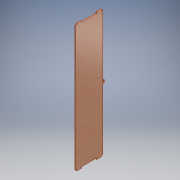
# Autodesk Inventor part: Frente_Controle
Saved by Autodesk Inventor 2017 (Build 210142000, 142)
## iProperties
Created: 2017-10-03
Part Number: Frente_Controle
Material: Wood (Oak)
Document SubType Name: Modeling
Designer: Felipe
Density: 0.76 g/cm^3
Appearance: White Oak - Natural Medium Gloss
Author: Felipe
Autodesk Inventor part; units mm, degrees
ref_plane "YZ Plane" through (0, 0, 0) normal (1, 0, 0) x (0, 1, 0)
ref_plane "XZ Plane" through (0, 0, 0) normal (0, 1, 0) x (-1, 0, 0)
sketch "Sketch1" plane through (0, 0, 0) normal (1, 0, 0) x (0, 1, 0)
  line L0 (0, 0) -> (195, 0) construction
  line L1 (195, 0) -> (195, -900)
  line L2 (195, -900) -> (0, -900) construction
  line L3 (0, -900) -> (0, 0)
  line L4 (195, -450) -> (0, -450) construction
  line L5 (186.046, 0) -> (151.046, 0) construction
  line L6 (151.046, 0) -> (151.046, 8.8542)
  line L7 (151.046, 8.8542) -> (186.046, 8.8542)
  line L8 (186.046, 8.8542) -> (186.046, 0)
  line L9 (43.046, 0) -> (8.046, 0) construction
  line L10 (8.046, 0) -> (8.046, 8.8542)
  line L11 (8.046, 8.8542) -> (43.046, 8.8542)
  line L12 (43.046, 8.8542) -> (43.046, 0)
  line L13 (151.046, 0) -> (43.046, 0)
  line L14 (8.046, 0) -> (0, 0)
  line L15 (186.046, 0) -> (195, 0)
  line L16 (0, -900) -> (195, -900) construction
  line L17 (186.046, -900) -> (151.046, -900) construction
  line L18 (151.046, -900) -> (151.046, -908.8542)
  line L19 (151.046, -908.8542) -> (186.046, -908.8542)
  line L20 (186.046, -908.8542) -> (186.046, -900)
  line L21 (43.046, -900) -> (8.046, -900) construction
  line L22 (8.046, -900) -> (8.046, -908.8542)
  line L23 (8.046, -908.8542) -> (43.046, -908.8542)
  line L24 (43.046, -908.8542) -> (43.046, -900)
  line L25 (151.046, -900) -> (43.046, -900)
  line L26 (8.046, -900) -> (0, -900)
  line L27 (186.046, -900) -> (195, -900)
  dimension "d0" = 900
  dimension "d1" = 195
  dimension "d2" = 35
  dimension "d3" = 108
  dimension "d4" = 8.046
  dimension "d5" = 8.954
  constraints: 56 end point, 8 symmetric about line, 6 parallel, 6 point on line, 4 collinear, 3 horizontal, 3 perpendicular, 2 midpoint
  measures "d0" distance of L0.end L1.end
  measures "d1" distance of L0.start L0.end
  measures "d2" distance of L6.end L7.end
  measures "d3" distance between parallel lines of L12 L6
  measures "d4" distance between parallel lines of L3 L10
  measures "d5" distance between parallel lines of L1 L8
extrude "Extrusion1" add sketch "Sketch1" along normal blind 6
ref_plane "Work Plane1" through (0, 43.046, -450) normal (0, 0, 1) x (1, 0, 0)
sketch "Sketch2" plane through (0, 43.046, -450) normal (0, 0, 1) x (1, 0, 0)
  line L0 (6, 143) -> (6, 151.954) projected
  circle A0 centre (11.3085, 152.954) radius 5
  circle A1 centre (11.3085, 152.954) radius 2.5
  line L1 (0, 151.954) -> (0, 143) projected
  line L2 (6, 151.954) -> (31.9194, 151.954) construction
  line L3 (6, 151.954) -> (6, 143) construction
  point P0 (0, -43.046)
  dimension "d11" = 5
  dimension "d12" = 10
  dimension "d13" = 1
  constraints: 2 centre point, 2 end point, 1 coincident, 1 horizontal
  measures "d11" diameter of A1
  measures "d12" diameter of A0
  measures "d13" distance from line of L2 A0.centre
extrude "Extrusion2" add sketch "Sketch2" along normal blind 15
body "Solid1"
